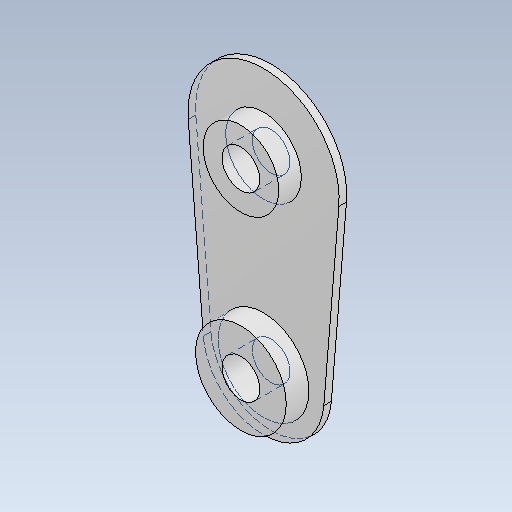
# Autodesk Inventor part: 揺動節抑え
Saved by Autodesk Inventor 2020 (Build 240168000, 168)
## iProperties
Created: 2020-10-27
Part Number: 揺動節抑え
Material: アルミニウム 2014-T4
Document SubType Name: Modeling
Designer: AA19065
Density: 2.8 g/cm^3
Appearance: サテン
Mass: 0.38813 g
Surface Area: 4.35352 cm^2
Volume: 0.138618 cm^3
Author: AA19065
Autodesk Inventor part; units mm, degrees
ref_plane "YZ Plane" through (0, 0, 0) normal (1, 0, 0) x (0, 1, 0)
ref_plane "XZ Plane" through (0, 0, 0) normal (0, 1, 0) x (-1, 0, 0)
ref_plane "XY Plane" through (0, 0, 0) normal (0, 0, 1) x (1, 0, 0)
sketch "スケッチ1" plane through (0, 0, 0) normal (0, 0, 1) x (1, 0, 0)
  circle A0 centre (0, 0) radius 5
  circle A1 centre (0, -25) radius 10 construction
  spline S0 degree 4 poles (38.5164, -45.3071) (38.2405, -45.4743) (37.8549, -45.7058) (37.3602, -45.9989) (36.7567, -46.3501) (36.3203, -46.6012) (35.8854, -46.8485) (35.4518, -47.0921) (35.0195, -47.332) (34.5884, -47.5683) (34.1585, -47.801) (33.7297, -48.0302) (33.3019, -48.256) (32.8751, -48.4784) (32.4492, -48.6974) (32.0242, -48.913) (31.6, -49.1254) (31.1766, -49.3346) (30.7539, -49.5405) (30.3319, -49.7433) (29.9104, -49.9429) (29.4896, -50.1394) (29.0693, -50.3329) (28.6495, -50.5233) (28.2302, -50.7106) (27.8112, -50.895) (27.3927, -51.0764) (26.9746, -51.2549) (26.5568, -51.4304) (26.1392, -51.603) (25.722, -51.7727) (25.3049, -51.9395) (24.8881, -52.1035) (24.4715, -52.2647) (24.0551, -52.423) (23.6388, -52.5785) (23.2226, -52.7313) (22.8066, -52.8812) (22.3906, -53.0284) (21.9747, -53.1728) (21.5589, -53.3145) (21.143, -53.4534) (20.7272, -53.5896) (20.3114, -53.723) (19.8956, -53.8538) (19.4798, -53.9818) (19.064, -54.1072) (18.6481, -54.2298) (18.2322, -54.3498) (17.8162, -54.4671) (17.4001, -54.5817) (16.984, -54.6936) (16.5678, -54.8028) (16.1515, -54.9094) (15.7351, -55.0133) (15.3186, -55.1146) (14.902, -55.2132) (14.4853, -55.3092) (14.0685, -55.4025) (13.6516, -55.4931) (13.2346, -55.5811) (12.8175, -55.6665) (12.4002, -55.7492) (11.9829, -55.8293) (11.5654, -55.9067) (11.1478, -55.9815) (10.7301, -56.0537) (10.3123, -56.1232) (9.8944, -56.19) (9.4764, -56.2543) (9.0583, -56.3159) (8.6401, -56.3748) (8.2218, -56.4311) (7.8034, -56.4848) (7.3849, -56.5359) (6.9663, -56.5843) (6.5476, -56.63) (6.1289, -56.6732) (5.7101, -56.7137) (5.2912, -56.7515) (4.8723, -56.7867) (4.4533, -56.8193) (4.0342, -56.8492) (3.6152, -56.8765) (3.1961, -56.9012) (2.7769, -56.9232) (2.3578, -56.9426) (1.9386, -56.9593) (1.5194, -56.9734) (1.1002, -56.9849) (0.6811, -56.9937) (0.2619, -56.9998) (-0.1572, -57.0034) (-0.5763, -57.0043) (-0.9954, -57.0025) (-1.4144, -56.9982) (-1.8334, -56.9911) (-2.2523, -56.9815) (-2.6711, -56.9692) (-3.0899, -56.9542) (-3.5086, -56.9366) (-3.9271, -56.9164) (-4.3456, -56.8935) (-4.764, -56.868) (-5.1823, -56.8399) (-5.6004, -56.8091) (-6.0185, -56.7757) (-6.4363, -56.7397) (-6.8541, -56.701) (-7.2717, -56.6597) (-7.6891, -56.6157) (-8.1064, -56.5691) (-8.5235, -56.5199) (-8.9404, -56.468) (-9.3572, -56.4135) (-9.7737, -56.3564) (-10.1901, -56.2966) (-10.6063, -56.2343) (-11.0222, -56.1692) (-11.438, -56.1016) (-11.8535, -56.0313) (-12.2688, -55.9584) (-12.6839, -55.8828) (-13.0988, -55.8046) (-13.5134, -55.7238) (-13.9278, -55.6404) (-14.342, -55.5543) (-14.7559, -55.4656) (-15.1696, -55.3743) (-15.5831, -55.2803) (-15.9963, -55.1837) (-16.4093, -55.0844) (-16.8221, -54.9826) (-17.2346, -54.878) (-17.6468, -54.7709) (-18.0589, -54.6611) (-18.4707, -54.5486) (-18.8822, -54.4336) (-19.2936, -54.3158) (-19.7047, -54.1954) (-20.1157, -54.0724) (-20.5264, -53.9467) (-20.9369, -53.8183) (-21.3473, -53.6872) (-21.7574, -53.5535) (-22.1674, -53.4171) (-22.5772, -53.278) (-22.9869, -53.1362) (-23.3965, -52.9916) (-23.8059, -52.8444) (-24.2153, -52.6945) (-24.6246, -52.5418) (-25.0338, -52.3863) (-25.4429, -52.2281) (-25.8521, -52.0672) (-26.2612, -51.9034) (-26.6704, -51.7368) (-27.0796, -51.5674) (-27.489, -51.3952) (-27.8984, -51.2201) (-28.308, -51.0421) (-28.7178, -50.8613) (-29.1278, -50.6775) (-29.538, -50.4907) (-29.9486, -50.3009) (-30.3595, -50.1082) (-30.7708, -49.9124) (-31.1826, -49.7135) (-31.5948, -49.5115) (-32.0076, -49.3063) (-32.4211, -49.0979) (-32.8352, -48.8863) (-33.2501, -48.6714) (-33.6658, -48.4531) (-34.0824, -48.2314) (-34.4999, -48.0062) (-34.9186, -47.7775) (-35.4969, -47.4575) (-35.9708, -47.1903) (-36.3399, -46.979) (-36.604, -46.8264) knots 0 0 0 0 0 0.015009 0.020983 0.026937 0.032872 0.038789 0.044688 0.05057 0.056436 0.062286 0.06812 0.073939 0.079743 0.085534 0.091311 0.097074 0.102825 0.108564 0.114291 0.120006 0.12571 0.131403 0.137086 0.142759 0.148421 0.154075 0.159719 0.165355 0.170982 0.1766 0.182211 0.187814 0.193409 0.198998 0.204579 0.210154 0.215722 0.221284 0.226839 0.232389 0.237934 0.243472 0.249006 0.254534 0.260058 0.265577 0.271091 0.276601 0.282106 0.287608 0.293105 0.298599 0.304089 0.309576 0.315059 0.320539 0.326015 0.331489 0.336959 0.342427 0.347893 0.353355 0.358815 0.364273 0.369729 0.375182 0.380633 0.386082 0.391529 0.396975 0.402419 0.407861 0.413301 0.41874 0.424177 0.429614 0.435048 0.440482 0.445915 0.451346 0.456777 0.462206 0.467635 0.473063 0.47849 0.483916 0.489342 0.494767 0.500192 0.505616 0.51104 0.516464 0.521888 0.527311 0.532734 0.538157 0.54358 0.549003 0.554426 0.559849 0.565273 0.570697 0.576121 0.581545 0.58697 0.592395 0.597821 0.603248 0.608675 0.614103 0.619532 0.624962 0.630393 0.635825 0.641257 0.646691 0.652127 0.657563 0.663001 0.668441 0.673881 0.679324 0.684768 0.690214 0.695662 0.701112 0.706564 0.712018 0.717474 0.722933 0.728394 0.733858 0.739324 0.744793 0.750265 0.755741 0.761219 0.766701 0.772186 0.777675 0.783167 0.788664 0.794164 0.799669 0.805178 0.810692 0.81621 0.821734 0.827263 0.832797 0.838337 0.843883 0.849434 0.854993 0.860558 0.86613 0.871709 0.877295 0.88289 0.888493 0.894104 0.899724 0.905353 0.910993 0.916642 0.922302 0.927972 0.933655 0.939349 0.945056 0.950775 0.956509 0.962257 0.968019 0.973798 0.979592 0.985404 1 1 1 1 1
  arc A2 (-34.6019, -43.3635) -> (-36.604, -46.8264) centre (-35.6029, -45.0949) ccw
  line L0 (-36.604, -46.8264) -> (-35.6029, -45.0949) construction
  line L1 (-34.6019, -43.3635) -> (-35.6029, -45.0949) construction
  arc A3 (9.9747, -25.7104) -> (36.4435, -41.8861) centre (27.3937, -26.9509) ccw
  arc A4 (-34.6019, -43.3635) -> (-9.8865, -26.5022) centre (-26.2949, -28.9953) ccw
  line L2 (-4.899, 1) -> (-9.798, -23) construction
  line L3 (4.899, 1) -> (9.798, -23) construction
  circle A5 centre (0, 0) radius 2.5
  circle A6 centre (0, 0) radius 1.25
  circle A7 centre (0, -12) radius 1.25
  circle A8 centre (0, -12) radius 3
  circle A9 centre (0, -12) radius 4.255 construction
  line L4 (-3.817, -10.1196) -> (-8.9705, -20.5808) construction
  line L5 (3.817, -10.1196) -> (8.9705, -20.5808) construction
  circle A10 centre (0, -25) radius 7.025 construction
  circle A11 centre (0, -12) radius 4
  line L6 (17.164, -48.1611) -> (13.7217, -46.1237)
  line L7 (13.7217, -46.1237) -> (15.7591, -42.6814)
  line L8 (15.7591, -42.6814) -> (19.2014, -44.7188)
  line L9 (19.2014, -44.7188) -> (17.164, -48.1611)
  line L10 (-17.2597, -45.3722) -> (-13.9841, -43.0765)
  line L11 (-13.9841, -43.0765) -> (-11.6884, -46.3522)
  line L12 (-11.6884, -46.3522) -> (-14.964, -48.6478)
  line L13 (-14.964, -48.6478) -> (-17.2597, -45.3722)
  line L14 (15.4429, -47.1424) -> (17.4802, -43.7001) construction
  line L15 (-15.6219, -44.2243) -> (-13.3262, -47.5) construction
  arc A12 (38.5164, -45.3071) -> (36.4435, -41.8861) centre (37.48, -43.5966) ccw
  line L16 (38.5164, -45.3071) -> (37.48, -43.5966) construction
  line L17 (36.4435, -41.8861) -> (37.48, -43.5966) construction
  line L18 (-5.2079, 2.2776) -> (-3.9861, -12.3333)
  line L19 (4.9826, -0.4167) -> (3.9861, -12.3333)
  point P0 (38.0735, -45.574)
  point P1 (37.6323, -45.8368)
  point P2 (37.1929, -46.0956)
  point P3 (36.755, -46.3505)
  point P4 (36.3186, -46.6016)
  point P5 (35.8837, -46.8488)
  point P6 (35.4502, -47.0924)
  point P7 (35.0179, -47.3322)
  point P8 (34.5869, -47.5685)
  point P9 (34.157, -47.8012)
  point P10 (33.7283, -48.0304)
  point P11 (33.3005, -48.2561)
  point P12 (32.8738, -48.4785)
  point P13 (32.4479, -48.6974)
  point P14 (32.023, -48.9131)
  point P15 (31.5988, -49.1254)
  point P16 (31.1754, -49.3346)
  point P17 (30.7527, -49.5405)
  point P18 (30.3307, -49.7432)
  point P19 (29.9093, -49.9428)
  point P20 (29.4885, -50.1393)
  point P21 (29.0683, -50.3328)
  point P22 (28.6485, -50.5231)
  point P23 (28.2292, -50.7105)
  point P24 (27.8103, -50.8948)
  point P25 (27.3918, -51.0762)
  point P26 (26.9737, -51.2547)
  point P27 (26.5559, -51.4302)
  point P28 (26.1384, -51.6028)
  point P29 (25.7211, -51.7725)
  point P30 (25.3041, -51.9393)
  point P31 (24.8874, -52.1033)
  point P32 (24.4708, -52.2644)
  point P33 (24.0544, -52.4227)
  point P34 (23.6381, -52.5782)
  point P35 (23.2219, -52.731)
  point P36 (22.8059, -52.8809)
  point P37 (22.39, -53.028)
  point P38 (21.9741, -53.1724)
  point P39 (21.5582, -53.3141)
  point P40 (21.1424, -53.453)
  point P41 (20.7266, -53.5892)
  point P42 (20.3109, -53.7226)
  point P43 (19.8951, -53.8534)
  point P44 (19.4793, -53.9814)
  point P45 (19.0635, -54.1068)
  point P46 (18.6476, -54.2294)
  point P47 (18.2317, -54.3494)
  point P48 (17.8157, -54.4666)
  point P49 (17.3997, -54.5812)
  point P50 (16.9836, -54.6931)
  point P51 (16.5674, -54.8024)
  point P52 (16.1511, -54.909)
  point P53 (15.7347, -55.0129)
  point P54 (15.3182, -55.1141)
  point P55 (14.9017, -55.2128)
  point P56 (14.485, -55.3087)
  point P57 (14.0682, -55.402)
  point P58 (13.6513, -55.4927)
  point P59 (13.2343, -55.5807)
  point P60 (12.8172, -55.666)
  point P61 (12.3999, -55.7487)
  point P62 (11.9826, -55.8288)
  point P63 (11.5651, -55.9062)
  point P64 (11.1476, -55.981)
  point P65 (10.7299, -56.0532)
  point P66 (10.3121, -56.1227)
  point P67 (9.8942, -56.1895)
  point P68 (9.4762, -56.2538)
  point P69 (9.0581, -56.3154)
  point P70 (8.6399, -56.3743)
  point P71 (8.2216, -56.4306)
  point P72 (7.8032, -56.4843)
  point P73 (7.3847, -56.5353)
  point P74 (6.9661, -56.5837)
  point P75 (6.5474, -56.6295)
  point P76 (6.1287, -56.6726)
  point P77 (5.7099, -56.7131)
  point P78 (5.2911, -56.751)
  point P79 (4.8721, -56.7862)
  point P80 (4.4532, -56.8187)
  point P81 (4.0341, -56.8487)
  point P82 (3.6151, -56.876)
  point P83 (3.196, -56.9006)
  point P84 (2.7768, -56.9226)
  point P85 (2.3577, -56.942)
  point P86 (1.9385, -56.9588)
  point P87 (1.5194, -56.9728)
  point P88 (1.1002, -56.9843)
  point P89 (0.681, -56.9931)
  point P90 (0.2619, -56.9993)
  point P91 (-0.1572, -57.0028)
  point P92 (-0.5763, -57.0037)
  point P93 (-0.9954, -57.002)
  point P94 (-1.4144, -56.9976)
  point P95 (-1.8334, -56.9906)
  point P96 (-2.2523, -56.9809)
  point P97 (-2.6711, -56.9686)
  point P98 (-3.0898, -56.9537)
  point P99 (-3.5085, -56.9361)
  point P100 (-3.9271, -56.9159)
  point P101 (-4.3456, -56.893)
  point P102 (-4.764, -56.8675)
  point P103 (-5.1822, -56.8394)
  point P104 (-5.6004, -56.8086)
  point P105 (-6.0184, -56.7752)
  point P106 (-6.4363, -56.7391)
  point P107 (-6.854, -56.7004)
  point P108 (-7.2716, -56.6591)
  point P109 (-7.689, -56.6152)
  point P110 (-8.1063, -56.5686)
  point P111 (-8.5234, -56.5194)
  point P112 (-8.9403, -56.4675)
  point P113 (-9.357, -56.413)
  point P114 (-9.7736, -56.3559)
  point P115 (-10.1899, -56.2961)
  point P116 (-10.6061, -56.2337)
  point P117 (-11.022, -56.1687)
  point P118 (-11.4378, -56.1011)
  point P119 (-11.8533, -56.0308)
  point P120 (-12.2686, -55.9579)
  point P121 (-12.6837, -55.8823)
  point P122 (-13.0985, -55.8041)
  point P123 (-13.5132, -55.7233)
  point P124 (-13.9276, -55.6399)
  point P125 (-14.3417, -55.5538)
  point P126 (-14.7557, -55.4651)
  point P127 (-15.1694, -55.3738)
  point P128 (-15.5828, -55.2798)
  point P129 (-15.996, -55.1832)
  point P130 (-16.409, -55.084)
  point P131 (-16.8217, -54.9821)
  point P132 (-17.2342, -54.8776)
  point P133 (-17.6465, -54.7704)
  point P134 (-18.0585, -54.6606)
  point P135 (-18.4703, -54.5482)
  point P136 (-18.8818, -54.4331)
  point P137 (-19.2932, -54.3154)
  point P138 (-19.7043, -54.195)
  point P139 (-20.1152, -54.0719)
  point P140 (-20.5259, -53.9462)
  point P141 (-20.9364, -53.8179)
  point P142 (-21.3468, -53.6868)
  point P143 (-21.7569, -53.5531)
  point P144 (-22.1669, -53.4167)
  point P145 (-22.5767, -53.2776)
  point P146 (-22.9864, -53.1358)
  point P147 (-23.3959, -52.9913)
  point P148 (-23.8053, -52.8441)
  point P149 (-24.2147, -52.6941)
  point P150 (-24.6239, -52.5414)
  point P151 (-25.0331, -52.386)
  point P152 (-25.4422, -52.2278)
  point P153 (-25.8514, -52.0669)
  point P154 (-26.2605, -51.9031)
  point P155 (-26.6697, -51.7366)
  point P156 (-27.0789, -51.5672)
  point P157 (-27.4882, -51.395)
  point P158 (-27.8976, -51.2199)
  point P159 (-28.3071, -51.0419)
  point P160 (-28.7169, -50.8611)
  point P161 (-29.1269, -50.6773)
  point P162 (-29.5371, -50.4905)
  point P163 (-29.9476, -50.3008)
  point P164 (-30.3585, -50.1081)
  point P165 (-30.7698, -49.9123)
  point P166 (-31.1815, -49.7134)
  point P167 (-31.5937, -49.5114)
  point P168 (-32.0065, -49.3063)
  point P169 (-32.4199, -49.0979)
  point P170 (-32.8339, -48.8863)
  point P171 (-33.2488, -48.6714)
  point P172 (-33.6644, -48.4532)
  point P173 (-34.081, -48.2315)
  point P174 (-34.4985, -48.0064)
  point P175 (-34.9171, -47.7778)
  point P176 (-35.3368, -47.5455)
  point P177 (-35.7578, -47.3096)
  point P178 (-36.1802, -47.0699)
  point P179 (-4.9826, -0.4167)
  dimension "d0" = 10
  dimension "d1" = 20
  dimension "d2" = 2
  dimension "d3" = 180
  dimension "d4" = 25
  dimension "d5" = 5
  dimension "d6" = 2.5
  dimension "d7" = 2.5
  dimension "d8" = 6
  dimension "d9" = 8.51
  dimension "d10" = 12
  dimension "d11" = 14.05
  dimension "d12" = 8
  dimension "d13" = 4
  dimension "d14" = 4
  dimension "d15" = 4
  dimension "d16" = 4
  dimension "d17" = 16.5967
  dimension "d18" = 17.4631
  dimension "d19" = 18.5967
  dimension "d20" = 19.4631
  dimension "d21" = 20
  dimension "d22" = 2
  dimension "d23" = 180
  dimension "d24" = 20
  constraints: 40 end point, 21 point on circle, 16 tangent, 13 centre point, 7 coincident, 4 midpoint, 4 parallel, 2 perpendicular, 2 point on line, 2 vertical alignment, 365 other
  measures "d0" diameter of A0
  measures "d1" diameter of A1
  measures "d2" radius of A2
  measures "d3" angle of L0 L1
  measures "d4" distance of A1.centre point (0, 0)
  measures "d5" diameter of A5
  measures "d6" diameter of A6
  measures "d7" diameter of A7
  measures "d8" diameter of A8
  measures "d9" diameter of A9
  measures "d10" distance of A7.centre point (0, 0)
  measures "d11" diameter of A10
  measures "d12" diameter of A11
  measures "d13" distance of L11.end L12.end
  measures "d14" distance of L6.start L6.end
  measures "d15" distance of L10.end L11.end
  measures "d16" distance of L6.end L7.end
  measures "d17" radius of A4
  measures "d18" radius of A3
  measures "d19" distance from line of A4.centre L10
  measures "d20" distance from line of A3.centre L8
  measures "d21" distance of L15.start L0.end
  measures "d22" radius of A12
  measures "d23" angle of L16 L17
  measures "d24" distance of L14.end L16.end
extrude "押し出し1" add sketch "スケッチ1" along normal blind 0.5 contours A0 | L19 A11 L18 A0 | A11
extrude "押し出し2" add sketch "スケッチ1" along normal blind 2 contours A5 | A8
equation "\"d4\" = d25"
equation "\"d6\" = d7"
equation "\"d25\" = 25"
